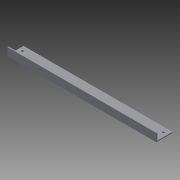
# Autodesk Inventor part: 2x2 angle horizontal
Saved by Autodesk Inventor 2015 SP1 (Build 190203100, 203)
## iProperties
Created: 2015-01-16
Part Number: 2x2 angle horizontal
Material: Generic
Document SubType Name: Modeling
Designer: 215152
Density: 1 g/cm^3
Appearance: Default
Author: 215152
Autodesk Inventor part; units mm, degrees
ref_plane "YZ Plane" through (0, 0, 0) normal (1, 0, 0) x (0, 1, 0)
ref_plane "XZ Plane" through (0, 0, 0) normal (0, 1, 0) x (-1, 0, 0)
ref_plane "XY Plane" through (0, 0, 0) normal (0, 0, 1) x (1, 0, 0)
sketch "Sketch1" plane through (0, 0, 0) normal (1, 0, 0) x (0, 1, 0)
  line L0 (0, 0) -> (3.175, 0)
  line L1 (3.175, 0) -> (3.175, -50.8)
  line L2 (3.175, -50.8) -> (0, -50.8)
  line L3 (0, -50.8) -> (0, 0)
  line L4 (0, 0) -> (50.8, 0)
  line L5 (50.8, 0) -> (50.8, -3.175)
  line L6 (50.8, -3.175) -> (0, -3.175)
  line L7 (0, -3.175) -> (0, 0)
  dimension "d0" = 3.175
  dimension "d1" = 50.8
  dimension "d2" = 50.8
  dimension "d3" = 3.175
  constraints: 16 end point, 4 parallel, 2 horizontal, 2 perpendicular
  measures "d0" distance of L1.end L2.end
  measures "d1" distance of L0.end L1.end
  measures "d2" distance of L5.end L6.end
  measures "d3" distance of L4.end L5.end
extrude "Extrusion1" add sketch "Sketch1" along normal blind 469.9
sketch "Sketch2" plane through (0, 0, -50.8) normal (0, -1, 0) x (1, 0, 0)
  line L0 (469.9, 50.8) -> (469.9, 0) projected
  line L1 (0, 50.8) -> (469.9, 50.8) projected
  line L2 (0, 50.8) -> (0, 0) projected
  line L3 (0, 0) -> (469.9, 0) projected
  point P0 (12.7, 41.275)
  point P1 (12.7, 15.875)
  point P2 (457.2, 41.275)
  point P3 (457.2, 15.875)
  dimension "d6" = 12.7
  dimension "d7" = 9.525
  dimension "d8" = 15.875
  dimension "d9" = 12.7
  dimension "d10" = 12.7
  dimension "d11" = 9.525
  dimension "d12" = 12.7
  dimension "d13" = 15.875
  measures "d6" distance from line of L0 point (457.2, 41.275)
  measures "d7" distance from line of L1 point (457.2, 41.275)
  measures "d8" distance from line of L3 point (457.2, 15.875)
  measures "d9" distance from line of L0 point (457.2, 15.875)
  measures "d10" distance from line of L2 point (12.7, 41.275)
  measures "d11" distance from line of L1 point (12.7, 41.275)
  measures "d12" distance from line of L2 point (12.7, 15.875)
  measures "d13" distance from line of L3 point (12.7, 15.875)
hole "Hole1" at (12.7, 0, -9.525) at (12.7, 0, -34.925) at (457.2, 0, -9.525) at (457.2, 0, -34.925) direction (0, 1, 0) diameter 6.35 end through all
sketch "Sketch3" plane through (0, 0, 0) normal (-1, 0, 0) x (0, 0, 1)
  line L0 (0, 0) -> (-50.8, 0) projected
  line L1 (0, 50.8) -> (0, 0) projected
  line L2 (-3.175, 50.8) -> (0, 50.8) projected
  line L3 (-3.175, 3.175) -> (-3.175, 50.8) projected
  line L4 (-50.8, 3.175) -> (-3.175, 3.175) projected
  line L5 (-50.8, 0) -> (-50.8, 3.175) projected
  line L6 (0, 50.8) -> (-3.175, 50.8)
  line L7 (-3.175, 50.8) -> (-3.175, 25.4)
  line L8 (-3.175, 25.4) -> (0, 25.4)
  line L9 (0, 25.4) -> (0, 50.8)
  dimension "d21" = 3.175
  dimension "d22" = 25.4
  constraints: 8 end point, 2 parallel, 1 horizontal, 1 perpendicular
  measures "d21" distance of L8.end L7.end
  measures "d22" distance of L7.end L6.end
extrude "Extrusion2" cut sketch "Sketch3" against normal blind 660.4 contours L8 L3 L2 L1
body "Solid1"
